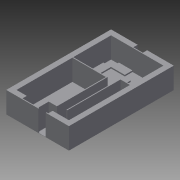
# Autodesk Inventor part: DelCo_2012_East_Structure
Saved by Autodesk Inventor 2014 (Build 180170000, 170)
## iProperties
Created: 2015-11-13
Part Number: DelCo_2012_East_Structure
Material: Generic
Document SubType Name: Modeling
Designer: jmw3
Density: 1 g/cm^3
Appearance: Default
Author: jmw3
Autodesk Inventor part; units mm, degrees
ref_plane "YZ Plane" through (0, 0, 0) normal (1, 0, 0) x (0, 1, 0)
ref_plane "XZ Plane" through (0, 0, 0) normal (0, 1, 0) x (-1, 0, 0)
ref_plane "XY Plane" through (0, 0, 0) normal (0, 0, 1) x (1, 0, 0)
sketch "Sketch1" plane through (0, 0, 0) normal (0, 1, 0) x (-1, 0, 0)
  line L0 (-3650, 6100) -> (-3650, -6100)
  line L1 (3650, -6100) -> (3650, 6100)
  line L2 (-3050, 5500) -> (-3050, -5500)
  line L3 (3050, -5500) -> (3050, 5500)
  line L4 (5110, 0) -> (-5110, 0) projected
  line L5 (0, -8540) -> (0, 8540) projected
  line L6 (-1150, 5500) -> (-1150, 6100)
  line L7 (1850, 5500) -> (1850, 6100)
  line L8 (550, -6100) -> (550, -5500)
  line L9 (-550, -6100) -> (-550, -5500)
  line L10 (-3650, -6100) -> (-550, -6100)
  line L11 (550, -6100) -> (3650, -6100)
  line L12 (-3050, -5500) -> (-550, -5500)
  line L13 (550, -5500) -> (3050, -5500)
  line L14 (3650, 6100) -> (1850, 6100)
  line L15 (-1150, 6100) -> (-3650, 6100)
  line L16 (3050, 5500) -> (1850, 5500)
  line L17 (-1150, 5500) -> (-3050, 5500)
  line L18 (3050, -1100) -> (-950, -1100)
  line L19 (-950, -1100) -> (-950, -1000)
  line L20 (-850, -1000) -> (3050, -1000)
  line L21 (3050, -1000) -> (3050, -1100)
  line L22 (1850, 6100) -> (-100, 6100)
  line L23 (-100, 6100) -> (-100, 6000)
  line L24 (1850, 6000) -> (1850, 6100)
  line L25 (0, 6000) -> (0, 4800)
  line L26 (100, 4700) -> (100, 6000)
  line L27 (-100, 6000) -> (0, 6000)
  line L28 (100, 6000) -> (1850, 6000)
  line L29 (-1150, 6100) -> (-950, 6100)
  line L30 (-950, 6100) -> (-950, 6000)
  line L31 (-950, 6000) -> (-1150, 6000)
  line L32 (-1150, 6000) -> (-1150, 6100)
  line L33 (0, 4800) -> (-950, 4800)
  line L34 (-950, 4800) -> (-950, 4700)
  line L35 (-850, 4700) -> (100, 4700)
  line L36 (100, 4700) -> (100, 4700)
  line L37 (-950, -1100) -> (-850, -1100)
  line L38 (-850, -1000) -> (-850, 4700)
  line L39 (-850, 4800) -> (-950, 4800)
  line L40 (-950, 4800) -> (-950, -1100)
  line L41 (-3050, -1700) -> (-1850, -1700)
  line L42 (-1850, -1700) -> (-1850, -1600)
  line L43 (-1950, -1600) -> (-3050, -1600)
  line L44 (-3050, -1600) -> (-3050, -1700)
  line L45 (-1850, -1700) -> (-1950, -1700)
  line L46 (-1950, -1600) -> (-1950, 4600)
  line L47 (-1950, 4600) -> (-1850, 4600)
  line L48 (-1850, 4600) -> (-1850, -1700)
  point P0 (0, 0)
  dimension "d0" = 7300
  dimension "d2" = 6100
  dimension "d5" = 1900
  dimension "d6" = 3000
  dimension "d7" = 2500
  dimension "d8" = 2500
  dimension "d9" = 12200
  dimension "d10" = 11000
  dimension "d11" = 100
  dimension "d12" = 4000
  dimension "d16" = 100
  dimension "d17" = 100
  dimension "d18" = 100
  dimension "d19" = 200
  dimension "d20" = 100
  dimension "d22" = 1200
  dimension "d23" = 6500
  dimension "d24" = 100
  dimension "d25" = 100
  dimension "d26" = 1200
  dimension "d27" = 3800
  dimension "d28" = 100
  dimension "d29" = 6300
  constraints: 94 end point, 27 parallel, 17 perpendicular, 11 horizontal, 8 collinear, 3 point on line, 4 other
  measures "d0" distance between parallel lines of L0 L1
  measures "d2" distance between parallel lines of L2 L3
  measures "d5" distance between parallel lines of L2 L6
  measures "d6" distance between parallel lines of L6 L7
  measures "d7" distance between parallel lines of L3 L8
  measures "d8" distance between parallel lines of L2 L9
  measures "d9" distance between parallel lines of L14 L11
  measures "d10" distance between parallel lines of L16 L13
  measures "d11" distance between parallel lines of L18 L20
  measures "d12" distance of L18.start L18.end
  measures "d16" distance between parallel lines of L23 L25
  measures "d17" distance between parallel lines of L25 L26
  measures "d18" distance between parallel lines of L22 L28
  measures "d19" distance between parallel lines of L32 L30
  measures "d20" distance between parallel lines of L35 L33
  measures "d22" distance between parallel lines of L28 L33
  measures "d23" distance between parallel lines of L16 L20
  measures "d24" distance between parallel lines of L38 L40
  measures "d25" distance between parallel lines of L41 L43
  measures "d26" distance between parallel lines of L2 L42
  measures "d27" distance between parallel lines of L12 L41
  measures "d28" distance between parallel lines of L48 L46
  measures "d29" distance between parallel lines of L41 L47
extrude "Extrusion1" add sketch "Sketch1" along normal blind 2438.4 contours L15 L6 L17 L2 L4 L0 | L4 L2 L12 L9 L10 L0 | L29 L30 L31 L6 | L43 L46 L4 L48 L42 L41 L2 | L46 L47 L48 L4 | L11 L8 L13 L3 L4 L1 | L4 L3 L16 L7 L14 L1 | L7 L28 L26 L35 L5 L22 | L3 L18 L5 L20 | L5 L27 L23 L22 | L5 L18 L19 L40 L4 L38 L20 | L4 L40 L34 L33 L5 L35 L38
sketch "Sketch2" plane through (0, 0, 0) normal (0, -1, 0) x (1, 0, 0)
  line L0 (-100, 6000) -> (-1850, 6000) projected
  line L1 (-100, 4700) -> (-100, 6000) projected
  line L2 (850, 4700) -> (-100, 4700) projected
  line L3 (850, -1000) -> (850, 4700) projected
  line L4 (-3050, -1000) -> (850, -1000) projected
  line L5 (-3050, 5500) -> (-3050, -1000) projected
  line L6 (-1850, 5500) -> (-3050, 5500) projected
  line L7 (-1850, 6000) -> (-1850, 5500) projected
  line L8 (-3650, 6100) -> (100, 6100) projected
  line L9 (-3650, -6100) -> (-3650, 6100) projected
  line L10 (-550, -6100) -> (-3650, -6100) projected
  line L11 (-550, -5500) -> (-550, -6100) projected
  line L12 (-3050, -5500) -> (-550, -5500) projected
  line L13 (-3050, -1100) -> (-3050, -5500) projected
  line L14 (950, -1100) -> (-3050, -1100) projected
  line L15 (950, 4800) -> (950, -1100) projected
  line L16 (0, 4800) -> (950, 4800) projected
  line L17 (0, 6000) -> (0, 4800) projected
  line L18 (100, 6000) -> (0, 6000) projected
  line L19 (100, 6100) -> (100, 6000) projected
  line L20 (-3650, 6100) -> (3650, 6100)
  line L21 (3650, 6100) -> (3650, -6100)
  line L22 (3650, -6100) -> (-3650, -6100)
  line L23 (-3650, -6100) -> (-3650, 6100)
  point P0 (0, 0)
  constraints: 8 end point, 2 parallel, 1 horizontal, 1 perpendicular
extrude "Extrusion2" add sketch "Sketch2" along normal blind 25.4 contours L1 L2 L3 L4 L5 L6 L7 L0 | L8 L19 L18 L17 L16 L15 L14 L13 L12 L11 L10 L9 | L20 L21 L22 L11 L12 L13 L14 L15 L16 L17 L18 L19
sketch "Sketch6" plane through (0, 0, 0) normal (0, 1, 0) x (1, 0, 0)
  line L0 (550, 6100) -> (550, 5500) projected
  line L1 (-550, 5500) -> (550, 5500)
  line L2 (550, 5500) -> (550, 5600)
  line L3 (550, 5600) -> (-550, 5600)
  line L4 (-550, 5600) -> (-550, 5500)
  point P0 (0, 0)
  dimension "d102" = 100
  constraints: 8 end point, 2 parallel, 1 horizontal, 1 perpendicular, 1 point on line
  measures "d102" distance between parallel lines of L1 L3
extrude "Extrusion6" add sketch "Sketch6" along normal up to surface (2438.4 mm away)
sketch "Sketch5" plane through (0, 0, 0) normal (0, 1, 0) x (1, 0, 0)
  line L0 (3050, 5500) -> (3050, 1700) projected
  line L1 (550, 5500) -> (3050, 5500) projected
  line L2 (-3050, 5500) -> (-550, 5500) projected
  line L3 (-3050, 1100) -> (-3050, 5500) projected
  line L4 (-2150, 5500) -> (-550, 5500)
  line L5 (-550, 5500) -> (-550, 4600)
  line L6 (-550, 4600) -> (-2150, 4600)
  line L7 (-2150, 4600) -> (-2150, 5500)
  line L8 (-3050, 4600) -> (-2150, 4600)
  line L9 (-2150, 4600) -> (-2150, 3000)
  line L10 (-2150, 3000) -> (-3050, 3000)
  line L11 (-3050, 3000) -> (-3050, 4600)
  line L12 (-350, 4400) -> (350, 4400)
  line L13 (350, 4400) -> (350, 3600)
  line L14 (350, 3600) -> (-350, 3600)
  line L15 (-350, 3600) -> (-350, 4400)
  line L16 (-2050, 3000) -> (-1250, 3000)
  line L17 (-1250, 3000) -> (-1250, 2300)
  line L18 (-1250, 2300) -> (-2050, 2300)
  line L19 (-2050, 2300) -> (-2050, 3000)
  point P0 (0, 0)
  dimension "d87" = 1600
  dimension "d88" = 900
  dimension "d89" = 900
  dimension "d90" = 1000
  dimension "d91" = 700
  dimension "d92" = 800
  dimension "d93" = 2700
  dimension "d94" = 1100
  dimension "d95" = 700
  dimension "d98" = 800
  dimension "d101" = 1600
  constraints: 32 end point, 8 parallel, 4 horizontal, 4 perpendicular, 3 collinear, 2 point on line
  measures "d87" distance between parallel lines of L10 L8
  measures "d88" distance between parallel lines of L2 L8
  measures "d89" distance between parallel lines of L3 L9
  measures "d90" distance between parallel lines of L3 L19
  measures "d91" distance between parallel lines of L16 L18
  measures "d92" distance between parallel lines of L19 L17
  measures "d93" distance between parallel lines of L0 L13
  measures "d94" distance between parallel lines of L1 L12
  measures "d95" distance between parallel lines of L13 L15
  measures "d98" distance between parallel lines of L12 L14
  measures "d101" distance between parallel lines of L7 L5
extrude "Furniture" add sketch "Sketch5" along normal blind 152.4 contours L2 L5 L6 L7 | L8 L9 L10 L3 | L12 L13 L14 L15 | L16 L17 L18 L19
sketch "Sketch4" plane through (0, 0, 0) normal (0, 1, 0) x (1, 0, 0)
  line L0 (-3050, 5500) -> (-550, 5500) projected
  line L1 (-3050, 1100) -> (-3050, 5500) projected
  line L2 (-2750, 5200) -> (-1750, 5200)
  line L3 (-1750, 5200) -> (-1750, 4000)
  line L4 (-1750, 4000) -> (-2750, 4000)
  line L5 (-2750, 4000) -> (-2750, 5200)
  line L6 (-2750, 3800) -> (-1750, 3800)
  line L7 (-1750, 3800) -> (-1750, 2600)
  line L8 (-1750, 2600) -> (-2750, 2600)
  line L9 (-2750, 2600) -> (-2750, 3800)
  point P0 (0, 0)
  dimension "d79" = 1000
  dimension "d80" = 1200
  dimension "d81" = 1200
  dimension "d82" = 200
  dimension "d83" = 300
  dimension "d84" = 300
  constraints: 16 end point, 4 parallel, 2 collinear, 2 horizontal, 2 perpendicular
  measures "d79" distance between parallel lines of L9 L7
  measures "d80" distance between parallel lines of L6 L8
  measures "d81" distance of L4.end L2.start
  measures "d82" distance between parallel lines of L6 L4
  measures "d83" distance between parallel lines of L0 L2
  measures "d84" distance between parallel lines of L1 L5
sketch "Sketch3" plane through (0, 0, 0) normal (0, 1, 0) x (1, 0, 0)
  line L0 (1950, -4600) -> (1950, 1600) projected
  line L1 (3050, 1700) -> (1850, 1700) projected
  line L2 (3050, 5500) -> (3050, 1700) projected
  line L3 (550, 5500) -> (3050, 5500) projected
  line L4 (-550, 6100) -> (550, 6100) projected
  line L5 (-3050, 5500) -> (-550, 5500) projected
  line L6 (-3050, 1100) -> (-3050, 5500) projected
  line L7 (950, 1100) -> (-3050, 1100) projected
  line L8 (950, -4800) -> (950, 1100) projected
  line L9 (0, -4800) -> (950, -4800) projected
  circle A0 centre (-1050, 3400) radius 152.4
  circle A1 centre (1050, 3400) radius 152.4
  line L10 (-1050, 3247.6) -> (-745.2, 3247.6)
  line L11 (-745.2, 3247.6) -> (-745.2, 3552.4)
  line L12 (-745.2, 3552.4) -> (-1050, 3552.4)
  line L13 (-1050, 3552.4) -> (-1050, 3247.6)
  line L14 (-1050, 3247.6) -> (-745.2, 3552.4) construction
  line L15 (-745.2, 3247.6) -> (-1050, 3552.4) construction
  line L16 (745.2, 3247.6) -> (1050, 3247.6)
  line L17 (1050, 3247.6) -> (1050, 3552.4)
  line L18 (1050, 3552.4) -> (745.2, 3552.4)
  line L19 (745.2, 3552.4) -> (745.2, 3247.6)
  line L20 (745.2, 3247.6) -> (1050, 3552.4) construction
  line L21 (1050, 3247.6) -> (745.2, 3552.4) construction
  line L22 (0, 8555.24) -> (0, -8631.44) projected
  line L23 (2297.6, 2147.6) -> (2602.4, 2147.6)
  line L24 (2602.4, 2147.6) -> (2602.4, 2452.4)
  line L25 (2602.4, 2452.4) -> (2297.6, 2452.4)
  line L26 (2297.6, 2452.4) -> (2297.6, 2147.6)
  line L27 (2297.6, 2147.6) -> (2602.4, 2452.4) construction
  line L28 (2602.4, 2147.6) -> (2297.6, 2452.4) construction
  line L29 (1251.4208, -2447.6) -> (1556.2208, -2447.6)
  line L30 (1251.4208, -2142.8) -> (1251.4208, -2447.6)
  line L31 (1251.4208, -2447.6) -> (1556.2208, -2142.8) construction
  line L32 (1556.2208, -2447.6) -> (1251.4208, -2142.8) construction
  line L33 (1251.4208, -2752.4) -> (1556.2208, -2752.4)
  line L34 (1556.2208, -2752.4) -> (1556.2208, -2447.6)
  line L35 (1556.2208, -2447.6) -> (1251.4208, -2447.6)
  line L36 (1251.4208, -2447.6) -> (1251.4208, -2752.4)
  line L37 (1251.4208, -2752.4) -> (1556.2208, -2447.6) construction
  line L38 (1556.2208, -2752.4) -> (1251.4208, -2447.6) construction
  line L39 (1251.4208, -2142.8) -> (1556.2208, -2447.6)
  ellipse E0 centre (1403.8208, 246) end of major axis (1403.8208, 500) minor radius 152.4
  line L40 (1850, 1700) -> (1950, 1600)
  ellipse E1 centre (2029.6051, 1520.3949) end of major axis (2209.2102, 1340.7898) minor radius 152.4
  line L41 (1403.8208, 500) -> (1403.8208, -8)
  line L42 (-3050, 5500) -> (-2150, 5500) projected
  line L43 (-3050, 1100) -> (-3050, 3000) projected
  line L44 (950, 1100) -> (-3050, 1100) projected
  line L45 (950, -4800) -> (950, 1100) projected
  line L46 (0, -4800) -> (950, -4800) projected
  line L47 (0, -6000) -> (0, -4800) projected
  line L48 (100, -6000) -> (0, -6000) projected
  line L49 (100, -6100) -> (100, -6000) projected
  line L50 (950, -6100) -> (100, -6100) projected
  line L51 (950, -6000) -> (950, -6100) projected
  line L52 (1150, -6000) -> (950, -6000) projected
  line L53 (1150, -5500) -> (1150, -6000) projected
  line L54 (3050, -5500) -> (1150, -5500) projected
  line L55 (3050, 1600) -> (3050, -5500) projected
  line L56 (1950, 1600) -> (3050, 1600) projected
  line L57 (1950, -4600) -> (1950, 1600) projected
  line L58 (1850, -4600) -> (1950, -4600) projected
  line L59 (1850, 1700) -> (1850, -4600) projected
  line L60 (3050, 1700) -> (1850, 1700) projected
  line L61 (3050, 5500) -> (3050, 1700) projected
  line L62 (372.6, -6252.4) -> (677.4, -6252.4)
  line L63 (372.6, -5947.6) -> (372.6, -6252.4)
  line L64 (372.6, -6252.4) -> (601.2, -6023.8) construction
  line L65 (677.4, -6252.4) -> (372.6, -5947.6) construction
  line L66 (372.6, -5947.6) -> (677.4, -6252.4)
  line L67 (-550, 5500) -> (-550, 4600) projected
  line L68 (-550, 4600) -> (-1750, 4600) projected
  line L69 (-1750, 4600) -> (-1750, 4000) projected
  line L70 (-1750, 4000) -> (-2150, 4000) projected
  line L71 (-2150, 4000) -> (-2150, 3800) projected
  line L72 (-2150, 3800) -> (-1750, 3800) projected
  line L73 (-1750, 3800) -> (-1750, 3000) projected
  line L74 (-1750, 3000) -> (-1250, 3000) projected
  line L75 (-1250, 3000) -> (-1250, 2300) projected
  line L76 (-1250, 2300) -> (-2050, 2300) projected
  line L77 (-2050, 2300) -> (-2050, 2600) projected
  line L78 (-2050, 2600) -> (-2750, 2600) projected
  line L79 (-2750, 2600) -> (-2750, 3000) projected
  line L80 (-2750, 3000) -> (-3050, 3000) projected
  line L81 (-550, 5500) -> (3050, 5500) projected
  line L82 (-2150, 5200) -> (-2150, 5500) projected
  line L83 (-3050, 4600) -> (-3050, 5500) projected
  line L84 (-3050, 4600) -> (-2750, 4600) projected
  line L85 (-2750, 4600) -> (-2750, 5200) projected
  line L86 (-2750, 5200) -> (-2150, 5200) projected
  point P0 (0, 0)
  point P1 (-897.6, 3400)
  point P2 (897.6, 3400)
  point P3 (0, 6100)
  point P4 (2450, 2300)
  point P5 (1403.8208, -2295.2)
  point P6 (1403.8208, -2600)
  point P7 (525, -6100)
  dimension "d73" = 152.4
  dimension "d74" = 254
  dimension "d75" = 254
  dimension "d76" = 152.4
  dimension "d34" = 2100
  dimension "d35" = 2000
  dimension "d36" = 2100
  dimension "d37" = 2000
  dimension "d38" = 304.8
  dimension "d39" = 304.8
  dimension "d40" = 2100
  dimension "d41" = 2100
  dimension "d43" = 304.8
  dimension "d44" = 304.8
  dimension "d45" = 304.8
  dimension "d51" = 600
  dimension "d52" = 600
  dimension "d53" = 304.8
  dimension "d54" = 304.8
  dimension "d56" = 2200
  dimension "d59" = 600
  dimension "d60" = 453.8208
  dimension "d61" = 453.8208
  dimension "d62" = 453.8208
  dimension "d63" = 304.8
  dimension "d65" = 304.8
  dimension "d66" = 304.8
  dimension "d107" = 304.8
  dimension "d108" = 304.8
  dimension "d109" = 45
  dimension "d110" = 152.4
  constraints: 73 end point, 16 midpoint, 8 parallel, 6 horizontal, 5 collinear, 4 perpendicular, 3 coincident, 3 point on line, 2 centre point, 1 symmetric about line, 1 vertical, 8 other
  measures "d34" distance from line of L3 point (1050, 3400)
  measures "d35" distance from line of L6 point (-1050, 3400)
  measures "d36" distance from line of L5 point (-1050, 3400)
  measures "d37" distance from line of L2 point (1050, 3400)
  measures "d38" diameter of A0
  measures "d39" diameter of A1
  measures "d40" distance from line of L3 point (897.6, 3400)
  measures "d41" distance from line of L5 point (-897.6, 3400)
  measures "d43" distance of L12.end L11.end
  measures "d44" distance between parallel lines of L10 L12
  measures "d45" distance of L18.end L17.end
  measures "d51" distance from line of L2 point (2450, 2300)
  measures "d52" distance from line of L1 point (2450, 2300)
  measures "d53" distance of L25.end L24.end
  measures "d54" distance between parallel lines of L23 L25
  measures "d56" distance from line of L9 point (1403.821, -2600)
  measures "d59" distance from line of L7 L41.start
  measures "d60" distance from line of L8 L41.start
  measures "d61" distance from line of L8 point (1403.821, -2295.2)
  measures "d62" distance from line of L8 point (1403.821, -2600)
  measures "d63" distance of L30.start L31.end
  measures "d65" distance of L35.end L34.end
  measures "d66" distance between parallel lines of L33 L35
  measures "d107" distance of L63.start L62.start
  measures "d108" distance of L62.start L62.end
  measures "d109" angle of L29 L39
  measures "d110" distance from line of L29 point (1403.821, -2295.2)
body "Solid1"
